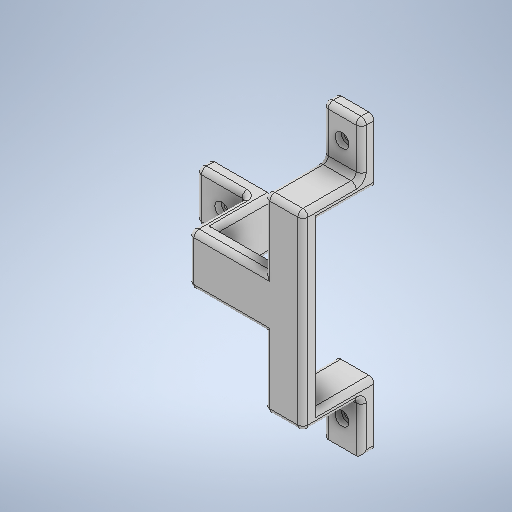
# Autodesk Inventor part: Battery mount
Saved by Autodesk Inventor 2025.1 (Build 291241000, 241)
## iProperties
Created: 2024-10-03
Part Number: Battery mount
Material: Generic
Document SubType Name: Modeling
Designer: bw1293
Density: 1 g/cm^3
Appearance: Default
Author: bw1293
Autodesk Inventor part; units mm, degrees
ref_plane "YZ Plane" through (0, 0, 0) normal (1, 0, 0) x (0, 1, 0)
ref_plane "XZ Plane" through (0, 0, 0) normal (0, 1, 0) x (-1, 0, 0)
ref_plane "XY Plane" through (0, 0, 0) normal (0, 0, 1) x (1, 0, 0)
sketch "Sketch1" plane through (0, 0, 0) normal (0, 0, 1) x (1, 0, 0)
  point P0 (0, 0)
sketch "Sketch2" plane through (0, 0, 0) normal (1, 0, 0) x (0, 1, 0)
  line L0 (37.5, -2.5) -> (-37.5, -2.5)
  line L1 (-37.5, -2.5) -> (-37.5, 2.5)
  line L2 (-37.5, 2.5) -> (37.5, 2.5)
  line L3 (37.5, 2.5) -> (37.5, -2.5)
  line L4 (37.5, -2.5) -> (-37.5, 2.5) construction
  line L5 (-37.5, -2.5) -> (37.5, 2.5) construction
  line L6 (37.5, -2.5) -> (32.5, -2.5)
  line L7 (32.5, -2.5) -> (32.5, -25.5)
  line L8 (32.5, -25.5) -> (37.5, -25.5)
  line L9 (37.5, -25.5) -> (37.5, -2.5)
  line L10 (-37.5, -2.5) -> (-32.5, -2.5)
  line L11 (-32.5, -2.5) -> (-32.5, -25.5)
  line L12 (-32.5, -25.5) -> (-37.5, -25.5)
  line L13 (-37.5, -25.5) -> (-37.5, -2.5)
  line L14 (37.5, -25.5) -> (57.5, -25.5)
  line L15 (57.5, -25.5) -> (57.5, -20.5)
  line L16 (57.5, -20.5) -> (37.5, -20.5)
  line L17 (37.5, -20.5) -> (37.5, -25.5)
  line L18 (-37.5, -25.5) -> (-57.5, -25.5)
  line L19 (-57.5, -25.5) -> (-57.5, -20.5)
  line L20 (-57.5, -20.5) -> (-37.5, -20.5)
  line L21 (-37.5, -20.5) -> (-37.5, -25.5)
  point P0 (0, 0)
  dimension "d0" = 75
  dimension "d1" = 5
  dimension "d2" = 5
  dimension "d3" = 23
  dimension "d4" = 5
  dimension "d5" = 23
  dimension "d6" = 20
  dimension "d7" = 5
  dimension "d8" = 20
  dimension "d9" = 5
  constraints: 44 end point, 10 parallel, 5 horizontal, 5 perpendicular, 2 midpoint
  measures "d0" distance of L1.end L2.end
  measures "d1" distance of L0.end L1.end
  measures "d2" distance of L8.end L7.end
  measures "d3" distance of L7.end L6.end
  measures "d4" distance of L11.end L12.end
  measures "d5" distance of L10.end L11.end
  measures "d6" distance of L16.end L15.end
  measures "d7" distance of L15.end L14.end
  measures "d8" distance of L19.end L20.end
  measures "d9" distance of L18.end L19.end
extrude "Extrusion1" add sketch "Sketch2" along normal blind 15
sketch "Sketch4" plane through (0, 37.5, -20.5) normal (0, 0, 1) x (1, 0, 0)
  line L0 (0, 0) -> (15, 0) projected
  line L1 (0, 20) -> (0, 0) projected
  line L2 (15, 0) -> (0, 20)
  line L3 (0, 20) -> (15, 20) projected
  line L4 (0, 20) -> (15, 20)
  line L5 (15, 20) -> (0, 0)
  circle A0 centre (7.5, 10) radius 1.5
  circle A1 centre (7.5, 10) radius 2.7
  point P0 (0, -37.5)
  dimension "d37" = 3
  dimension "d38" = 5.4
  constraints: 6 end point, 2 centre point, 1 coincident, 1 collinear, 1 midpoint
  measures "d37" diameter of A0
  measures "d38" diameter of A1
hole "Hole4" at (7.5, 47.5, -20.5) direction (0, 0, -1) diameter 3 end through all counterbore diameter 5.4 counterbore depth 2.4
sketch "Sketch5" plane through (0, -57.5, -20.5) normal (0, 0, 1) x (1, 0, 0)
  line L0 (0, 20) -> (15, 20) projected
  line L1 (0, 0) -> (0, 25) projected
  line L2 (0, 0) -> (15, 0) projected
  line L3 (0, 0) -> (15, 0)
  line L4 (0, 95) -> (0, 20) projected
  circle A0 centre (7.5, 10) radius 1.5
  point P0 (0, 57.5)
  dimension "d46" = 3
  constraints: 2 end point, 1 centre point, 1 collinear
  measures "d46" diameter of A0
hole "Hole5" at (7.5, -47.5, -20.5) direction (0, 0, -1) diameter 3 end through all counterbore diameter 5.4 counterbore depth 2.4
sketch "Sketch6" plane through (0, 0, 0) normal (-1, 0, 0) x (0, 0, 1)
  line L0 (-2.5, 10) -> (2.5, 10)
  line L1 (2.5, 10) -> (2.5, -10)
  line L2 (2.5, -10) -> (-2.5, -10)
  line L3 (-2.5, -10) -> (-2.5, 10)
  line L4 (-2.5, 10) -> (2.5, -10) construction
  line L5 (2.5, 10) -> (-2.5, -10) construction
  point P0 (0, 0)
  dimension "d54" = 5
  dimension "d55" = 20
  constraints: 12 end point, 2 midpoint, 2 parallel, 1 horizontal, 1 perpendicular
  measures "d54" distance of L1.end L2.end
  measures "d55" distance of L0.end L1.end
extrude "Extrusion2" add sketch "Sketch6" along normal blind 30
sketch "Sketch7" plane through (0, 10, 2.5) normal (0, 1, 0) x (1, 0, 0)
  line L0 (0, 5) -> (-30, 5) projected
  line L1 (-30, 5) -> (-25, 5)
  line L2 (-25, 5) -> (-25, 28)
  line L3 (-25, 28) -> (-30, 28)
  line L4 (-30, 28) -> (-30, 5)
  point P0 (0, 2.5)
  dimension "d58" = 5
  dimension "d59" = 23
  constraints: 8 end point, 2 parallel, 1 horizontal, 1 perpendicular
  measures "d58" distance of L3.end L2.end
  measures "d59" distance of L2.end L1.end
extrude "Extrusion3" add sketch "Sketch7" against normal blind 20
sketch "Sketch8" plane through (-30, 0, 0) normal (-1, 0, 0) x (0, 0, 1)
  line L0 (-2.5, 10) -> (-25.5, 10) projected
  line L1 (2.5, -10) -> (-25.5, -10) projected
  line L2 (-25.5, 10) -> (-20.5, 10)
  line L3 (-20.5, 10) -> (-20.5, -10)
  line L4 (-20.5, -10) -> (-25.5, -10)
  line L5 (-25.5, -10) -> (-25.5, 10)
  point P0 (0, 0)
  dimension "d62" = 5
  constraints: 8 end point, 2 parallel, 1 horizontal, 1 perpendicular, 1 point on line
  measures "d62" distance of L3.end L4.end
extrude "Extrusion4" add sketch "Sketch8" along normal blind 20
sketch "Sketch9" plane through (-30, -10, -20.5) normal (0, 0, 1) x (1, 0, 0)
  line L0 (5, 0) -> (-20, 0) projected
  line L1 (0, 0) -> (0, 20) projected
  line L2 (-20, 0) -> (0, 20)
  line L3 (0, 20) -> (0, 0)
  line L4 (0, 0) -> (-20, 20)
  circle A0 centre (-10, 10) radius 1.5
  point P0 (30, 10)
  dimension "d65" = 3
  constraints: 6 end point, 1 centre point, 1 midpoint, 1 perpendicular, 1 vertical
  measures "d65" diameter of A0
hole "Hole6" at (-40, 0, -20.5) direction (0, 0, -1) diameter 3 end through all counterbore diameter 5.4 counterbore depth 2.4
fillet "Fillet1" radius 2 37 edges at (15, 37.5, -9) (0, 37.5, -9) (0, 47.5, -20.5) (15, 47.5, -20.5) (7.5, 57.5, -20.5) (0, 57.5, -23) (15, 57.5, -23) (7.5, 37.5, -20.5) (15, 0, 2.5) (0, 23.75, 2.5) (0, -23.75, 2.5) (-15, 10, 2.5) (-15, -10, 2.5) (7.5, -37.5, 2.5) (7.5, 37.5, 2.5) (-30, 0, 2.5) (0, -37.5, -9) (7.5, -37.5, -20.5) (15, -37.5, -9) (0, -57.5, -23) (15, -57.5, -23) (15, -47.5, -20.5) (0, -47.5, -20.5) (0, -32.5, -14) (15, -32.5, -14) (0, 32.5, -14) (15, 32.5, -14) (-40, -10, -20.5) (-50, -10, -23) (-50, 0, -20.5) (-25, -10, -14) (-30, -10, -9) (-30, 10, -9) (-30, 0, -20.5) (-40, 10, -20.5) (-50, 10, -23) (-25, 10, -14)
body "Solid1"
